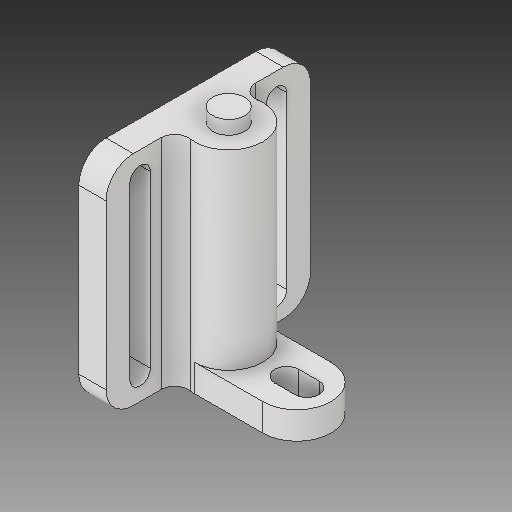
# Autodesk Inventor part: Pok Mk3 Yaw Motor Support
Saved by Autodesk Inventor 2018.2 (Build 222227000, 227)
## iProperties
Created: 2018-02-27
Part Number: Pok Mk3 Yaw Motor Support
Material: ABS Plastic
Document SubType Name: Modeling
Designer: Moochster
Density: 1.06 g/cm^3
Appearance: Smooth - White
Mass: 6.08773 g
Surface Area: 33.1126 cm^2
Volume: 5.74314 cm^3
Author: Moochster
Autodesk Inventor part; units mm, degrees
ref_plane "XZ Plane" through (0, 0, 0) normal (0, 1, 0) x (-1, 0, 0)
sketch "Sketch1" plane through (0, 0, 0) normal (0, 1, 0) x (-1, 0, 0)
  circle A0 centre (0, 0) radius 2.35
  circle A1 centre (0, 0) radius 5
  line L0 (0, 5) -> (-10, 5)
  arc A2 (-10, 5) -> (-10, -5) centre (-10, 0) ccw
  line L1 (-10, -5) -> (0, -5)
  line L2 (-8.5, 0) -> (-11.5, 0) construction
  line L3 (-8.5, 1.75) -> (-11.5, 1.75)
  line L4 (-11.5, -1.75) -> (-8.5, -1.75)
  arc A3 (-8.5, -1.75) -> (-8.5, 1.75) centre (-8.5, 0) ccw
  arc A4 (-11.5, 1.75) -> (-11.5, -1.75) centre (-11.5, 0) ccw
  dimension "d0" = 4.7
  dimension "d1" = 10
  dimension "d36" = 5
  dimension "d37" = 1.75
  dimension "d38" = 10
  dimension "d39" = 3
  constraints: 12 end point, 8 point on circle, 8 tangent, 5 centre point, 2 coincident, 2 horizontal, 1 midpoint, 1 parallel
  measures "d0" diameter of A0
  measures "d1" diameter of A1
  measures "d36" radius of A2
  measures "d37" radius of A4
  measures "d38" distance of point (0, 0) A2.centre
  measures "d39" distance of L2.start L2.end
extrude "Extrusion1" add sketch "Sketch1" against normal blind 2 and the other way blind 2 contours A0 | A1 | A1 L1 A2 L0
extrude "Extrusion2" add sketch "Sketch1" along normal blind 30 contours A1
extrude "Extrusion3" add sketch "Sketch1" along normal blind 32 contours A0
ref_plane "Work Plane1" through (-5, 0, 0) normal (1, 0, 0) x (0, 1, 0)
ref_plane "Work Plane2" through (-7, 0, 0) normal (1, 0, 0) x (0, 1, 0)
sketch "Sketch2" plane through (-7, 0, 0) normal (1, 0, 0) x (0, 1, 0)
  line L0 (30, -15) -> (-2, -15)
  line L1 (-2, 15) -> (30, 15)
  line L2 (30, 15) -> (30, -15)
  line L3 (30, -5) -> (30, 5) projected
  line L4 (2, -5) -> (-2, -5) projected
  line L5 (-2, 5) -> (-2, -5) projected
  line L6 (2, 5) -> (-2, 5) projected
  line L7 (2, -5) -> (2, 5) projected
  line L8 (-2, -15) -> (-2, 15)
  point P0 (0, 0)
  dimension "d11" = 30
  dimension "d12" = 15
  constraints: 8 end point, 1 horizontal, 1 parallel, 1 vertical, 1 vertical alignment
  measures "d11" distance between parallel lines of L0 L1
  measures "d12" distance from line of point (0, 0) L1
extrude "Extrusion4" add sketch "Sketch2" along normal blind 4
sketch "Sketch4" plane through (-7, 0, 0) normal (-1, 0, 0) x (0, 0, 1)
  line L0 (10, 26.5) -> (10, 1.5) construction
  line L1 (8.5, 26.5) -> (8.5, 1.5)
  line L2 (11.5, 1.5) -> (11.5, 26.5)
  arc A0 (11.5, 26.5) -> (8.5, 26.5) centre (10, 26.5) ccw
  arc A1 (8.5, 1.5) -> (11.5, 1.5) centre (10, 1.5) ccw
  line L3 (-10, 26.5) -> (-10, 1.5) construction
  line L4 (-11.5, 26.5) -> (-11.5, 1.5)
  line L5 (-8.5, 1.5) -> (-8.5, 26.5)
  arc A2 (-8.5, 26.5) -> (-11.5, 26.5) centre (-10, 26.5) ccw
  arc A3 (-11.5, 1.5) -> (-8.5, 1.5) centre (-10, 1.5) ccw
  line L6 (15, -2) -> (15, 30) projected
  line L7 (10, 14) -> (-10, 14) construction
  point P0 (0, 0)
  point P1 (15, 14)
  point P2 (0, 14)
  dimension "d30" = 20
  dimension "d31" = 1.5
  dimension "d32" = 25
  constraints: 18 end point, 8 point on circle, 8 tangent, 4 centre point, 4 midpoint, 3 horizontal alignment, 3 parallel, 1 equal radius, 1 horizontal, 1 vertical, 1 vertical alignment
  measures "d30" distance between parallel lines of L3 L0
  measures "d31" radius of A1
  measures "d32" distance of L0.start L0.end
extrude "Extrusion5" cut sketch "Sketch4" against normal up to surface (4 mm away)
fillet "Fillet1" radius 2 2 edges at (-3, 14, -4) (-3, 14, 4)
fillet "Fillet2" radius 4 4 edges at (-5, 30, 15) (-5, -2, 15) (-5, -2, -15) (-5, 30, -15)
body "Solid1"
